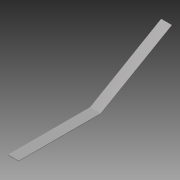
# Autodesk Inventor part: slats
Saved by Autodesk Inventor 2013 (Build 170138000, 138)
## iProperties
Created: 2012-12-18
Part Number: slats
Material: Steel, Carbon
Document SubType Name: Sheet Metal
Designer: istvan.burbank
Density: 7.87 g/cm^3
Sheet Metal Rule: Default
Flat Pattern Width: 7.62 cm
Flat Pattern Length: 117.087 cm
Flat Pattern Area: 892.199 cm^2
Sheet Metal Width: 3.000 in
Sheet Metal Length: 46.097 in
Sheet Metal Area: 138.291 in^2
Author: istvan.burbank
Autodesk Inventor part; units mm, degrees
ref_plane "YZ Plane" through (0, 0, 0) normal (1, 0, 0) x (0, 1, 0)
ref_plane "XZ Plane" through (0, 0, 0) normal (0, 1, 0) x (-1, 0, 0)
ref_plane "XY Plane" through (0, 0, 0) normal (0, 0, 1) x (1, 0, 0)
sketch "Sketch1" plane through (0, 0, 0) normal (0, 1, 0) x (-1, 0, 0)
  line L0 (0, 0) -> (76.2, 0)
  line L1 (76.2, 0) -> (76.2, 1828.8)
  line L2 (76.2, 1828.8) -> (0, 1828.8)
  line L3 (0, 1828.8) -> (0, 0)
  dimension "d0" = 76.2
  dimension "d1" = 1828.8
  measures "d0" distance of L2.end L1.end
  measures "d1" distance of L1.end L0.end
extrude "Plate1" add sketch "Sketch1" against normal blind 3.175
sketch "Sketch2" plane through (0, 0, 0) normal (0, 1, 0) x (1, 0, 0)
  line L0 (0, 0) -> (-76.2, 0) projected
  line L1 (-76.2, 0) -> (-76.2, -1828.8) projected
  line L2 (-76.2, -1828.8) -> (0, -1828.8) projected
  line L3 (0, -1828.8) -> (0, 0) projected
  line L4 (-76.2, -914.4) -> (0, -914.4)
  dimension "d3" = 914.4
  dimension "d4" = 914.4
  constraints: 2 end point, 2 midpoint, 1 perpendicular
  measures "d3" distance between parallel lines of L0 L4
  measures "d4" distance between parallel lines of L2 L4
fold "Fold1" angle 30 bend radius 3.175 thickness 3.175 k factor 0.44 line from (-76.2, 0, 914.4) to (0, 0, 914.4) line at bend centre moving side (0, 0, -1) folds toward (0, 1, 0)
sketch "Sketch3" plane through (0, 0.4254, 914.0094) normal (1, 0, 0) x (0, 0.5, -0.8660254)
  line L0 (0, -3.175) -> (913.2031, -3.175) projected
  line L1 (913.2031, 0) -> (913.2031, -3.175) projected
  line L2 (0, 0) -> (913.2031, 0) projected
  line L3 (-3.175, -2.3243) -> (-1.5875, 0.4254) projected
  line L4 (-792.4445, 457.0269) -> (-1.5875, 0.4254) projected
  line L5 (-792.4445, 457.0269) -> (-794.032, 454.2773) projected
  line L6 (-794.032, 454.2773) -> (-3.175, -2.3243) projected
  line L7 (-507.5504, 292.5432) -> (584.2356, 0)
  line L8 (-507.5504, 292.5432) -> (-509.1379, 289.7935)
  line L9 (584.2356, 0) -> (584.2356, -3.175)
  point P0 (791.3427, -457.3731)
  dimension "d11" = 1130.3
  dimension "d12" = 584.2356
  dimension "d13" = 584.2356
  constraints: 6 end point, 4 point on line, 2 perpendicular
  measures "d11" distance of L7.start L7.end
  measures "d12" distance of L7.start L3.end
  measures "d13" distance of L7.end L2.start
extrude "Extrusion1" cut sketch "Sketch3" against normal through all contours L9 L2 L1 L0 | L6 L5 L4 L8
equation "\"d3\" = d4"
equation "\"d5\" = BendReliefWidth"
equation "\"d6\" = BendReliefDepth"
equation "\"d7\" = MinimumRemnant"
equation "\"d8\" = BendRadius"
equation "\"d10\" = BendRadius"
equation "\"d12\" = d13"
equation "\"BendRadius\" = Thickness"
equation "\"BendReliefWidth\" = Thickness"
equation "\"BendReliefDepth\" = 0.5 * Thickness"
equation "\"CornerReliefSize\" = 4 * Thickness"
equation "\"MinimumRemnant\" = 2 * Thickness"
equation "\"TransitionRadius\" = BendRadius"
equation "\"JacobiRadiusSize\" = BendRadius"
equation "\"GapSize\" = Thickness"
equation "\"d2\" = BendRadius"
equation "\"Thickness\" = 3.175"
body "Solid1"
